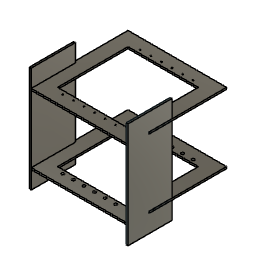
ionenantrieb v1 v1 (Autodesk Fusion 360 design; units mm, degrees)
Autodesk Fusion 360 part; units mm, degrees
sketch "Skizze1" plane through (0, 0, 0) normal (0, 0, 1) x (1, 0, 0)
  line L0 (0, 0) -> (100, 0)
  line L1 (100, 0) -> (100, 100)
  line L2 (100, 100) -> (0, 100)
  line L3 (0, 100) -> (0, 0)
  line L4 (-17.4, -20) -> (120, -20)
  line L5 (120, -20) -> (120, 120)
  line L6 (120, 120) -> (-20, 120)
  line L7 (-20, 120) -> (-20, 10)
  line L8 (-20, 10) -> (-17.4, 10)
  line L9 (-17.4, 10) -> (-17.4, -20)
  line L10 (50, 0) -> (50, 5)
  line L11 (117.4, 10) -> (117.4, -20)
  line L12 (120, 10) -> (117.4, 10)
  dimension "d1" = 100
  dimension "d2" = 100
  dimension "d4" = 2.6
  dimension "d5" = 30
  constraint horizontal L0
  constraint vertical L1
  constraint horizontal L2
  constraint vertical L3
  constraint coincident L0.start L3.end
  constraint perpendicular L7 L8
  constraint perpendicular L4 L9
  constraint parallel L0 L4
  constraint parallel L1 L5
  constraint parallel L2 L6
  constraint parallel L3 L7
  constraint midpoint L0 L10.start
  constraint perpendicular L0 L10
  constraint symmetric L7.end L10 L12.start
  constraint symmetric L8.end L10 L11.start
  constraint symmetric L4.start L10 L11.end
  measures "d1" distance of L1.end L2.end
  measures "d2" distance of L0.start L2.end
  measures "d4" distance of L7.end L8.end
  measures "d5" distance of L8.end L4.start
extrude "Extrusion1" add sketch "Skizze1" along normal blind 2.5 contours L4 L5 L6 L7 L8 L9 L11 L12 makes body 1
sketch "Skizze2" plane through (-17.4, 0, 0) normal (-1, 0, 0) x (0, -1, 0)
  line L0 (-10, 0) -> (20, 0)
  line L1 (20, 0) -> (20, 2.5)
  line L2 (20, 2.5) -> (-10, 2.5)
  line L3 (-10, 2.5) -> (-10, 0)
  line L4 (20, -25) -> (-42.7296, -25)
  line L5 (-42.7296, 125) -> (20, 125)
  line L6 (20, 125) -> (20, -25)
  line L7 (-10, 2.5) -> (-42.7296, 2.5)
  line L8 (-10, 0) -> (-42.7296, 0)
  line L9 (-10, 0) -> (-10, 2.5)
  line L10 (-42.7296, 50) -> (-35, 50)
  line L11 (-10, 100) -> (-42.7296, 100)
  line L12 (-10, 97.5) -> (-42.7296, 97.5)
  line L13 (-10, 100) -> (-10, 97.5)
  line L14 (-42.7296, -25) -> (-42.7296, 0)
  line L15 (-42.7296, 2.5) -> (-42.7296, 97.5)
  line L16 (-42.7296, 100) -> (-42.7296, 125)
  dimension "d8" = 150
  dimension "d9" = 25
  constraint horizontal L4
  constraint vertical L14
  constraint horizontal L5
  constraint vertical L6
  constraint coincident L2.end L3.start
  constraint coincident L7.end L14
  constraint perpendicular L7 L14
  constraint coincident L0.start L3.end
  constraint perpendicular L8 L14
  constraint perpendicular L10 L14
  constraint symmetric L2.end L10 L12.start
  constraint symmetric L7.end L10 L12.end
  constraint symmetric L0.start L10 L11.start
  constraint symmetric L8.end L10 L11.end
  constraint collinear L14 L15
  constraint coincident L10.start L14
  constraint collinear L15 L16
  measures "d8" distance of L4.end L5.start
  measures "d9" distance of L4 L8
extrude "Extrusion2" add sketch "Skizze2" along normal blind 2.5 separate body makes body 2
ref_plane "Arbeitsebene1" through (-18.65, 11.3648, 50) normal (0, 0, -1) x (0, -1, 0)
mirror "Spiegeln1" about plane through (-18.65, 11.3648, 50) normal (0, 0, -1) of bodies 1 makes body 3
ref_plane "Arbeitsebene2" through (50, 65, 98.75) normal (1, 0, 0) x (0, 1, 0)
mirror "Spiegeln2" about plane through (50, 65, 98.75) normal (1, 0, 0) of bodies 2 makes body 4
sketch "Skizze3" plane through (0, 0, 2.5) normal (0, 0, 1) x (-1, 0, 0)
  line L0 (0, 0) -> (0, -100)
  line L1 (0, -100) -> (-100, -100)
  line L2 (-100, -100) -> (-100, 0)
  line L3 (-100, 0) -> (0, 0)
  line L4 (-120, -120) -> (20, -120)
  line L5 (20, -120) -> (20, -10)
  line L6 (20, -10) -> (17.4, -10)
  line L7 (17.4, -10) -> (17.4, 20)
  line L8 (17.4, 20) -> (-117.4, 20)
  line L9 (-117.4, 20) -> (-117.4, -10)
  line L10 (-117.4, -10) -> (-120, -10)
  line L11 (-120, -10) -> (-120, -120)
  circle A0 centre (-12.5, -105) radius 2
  circle A1 centre (-27.5, -105) radius 2
  circle A2 centre (-42.5, -105) radius 2
  circle A3 centre (-57.5, -105) radius 2
  circle A4 centre (-72.5, -105) radius 2
  line L12 (0, -50) -> (-0.7928, -50)
  circle A5 centre (-27.5, 5) radius 2
  circle A6 centre (-72.5, 5) radius 2
  circle A7 centre (-42.5, 5) radius 2
  circle A8 centre (-57.5, 5) radius 2
  circle A9 centre (-12.5, 5) radius 2
  circle A10 centre (-87.5, -105) radius 2
  circle A11 centre (-87.5, 5) radius 2
  point P0 (-87.5, 5)
  dimension "d16" = 4
  dimension "d17" = 5
  dimension "d18" = 12.5
  dimension "d21" = 75
  dimension "d22" = 0
  constraint midpoint L0 L12.start
  constraint perpendicular L0 L12
  constraint symmetric A0 L12 A9
  constraint symmetric A1 L12 A5
  constraint symmetric A2 L12 A7
  constraint symmetric A3 L12 A8
  constraint symmetric A4 L12 A6
  constraint symmetric L12 A10.centre P0
  constraint symmetric L12 A10 A11
  measures "d16" diameter of A0
  measures "d17" distance of L1 A0.centre
  measures "d18" distance of L0 A0.centre
extrude "Extrusion3" cut sketch "Skizze3" against normal blind 2.5 contours A0 | A1 | A2 | A3 | A4 | A5 | A6 | A7 | A8 | A9 | A10 | A11 bodies 1
sketch "Skizze4" plane through (0, 0, 100) normal (0, 0, 1) x (-1, 0, 0)
  line L0 (0, 0) -> (0, -100)
  line L1 (0, -100) -> (-100, -100)
  line L2 (-100, -100) -> (-100, 0)
  line L3 (-100, 0) -> (0, 0)
  line L4 (-120, -120) -> (20, -120)
  line L5 (20, -120) -> (20, -10)
  line L6 (20, -10) -> (17.4, -10)
  line L7 (17.4, -10) -> (17.4, 20)
  line L8 (17.4, 20) -> (-117.4, 20)
  line L9 (-117.4, 20) -> (-117.4, -10)
  line L10 (-117.4, -10) -> (-120, -10)
  line L11 (-120, -10) -> (-120, -120)
  circle A0 centre (-12.5, -105) radius 1
  circle A1 centre (-27.5, -105) radius 1
  circle A2 centre (-42.5, -105) radius 1
  circle A3 centre (-57.5, -105) radius 1
  circle A4 centre (-72.5, -105) radius 1
  line L12 (0, -50) -> (-0.625, -50)
  circle A5 centre (-27.5, 5) radius 1
  circle A6 centre (-72.5, 5) radius 1
  circle A7 centre (-42.5, 5) radius 1
  circle A8 centre (-12.5, 5) radius 1
  circle A9 centre (-57.5, 5) radius 1
  circle A10 centre (-87.5, -105) radius 1
  circle A11 centre (-87.5, 5) radius 1
  dimension "d25" = 2
  dimension "d26" = 5
  dimension "d27" = 12.5
  dimension "d30" = 75
  dimension "d31" = 0
  constraint midpoint L0 L12.start
  constraint perpendicular L0 L12
  constraint symmetric A0 L12 A8
  constraint symmetric A1 L12 A5
  constraint symmetric A2 L12 A7
  constraint symmetric A3 L12 A9
  constraint symmetric A4 L12 A6
  constraint symmetric L12 A10 A11
  measures "d25" diameter of A0
  measures "d26" distance of L1 A0.centre
  measures "d27" distance of L0 A0.centre
extrude "Extrusion4" cut sketch "Skizze4" against normal blind 2.5 contours A0 | A1 | A2 | A3 | A4 | A5 | A6 | A7 | A8 | A9 | A10 | A11 bodies 3
sketch "Skizze5" plane through (117.4, 0, 0) normal (-1, 0, 0) x (0, -1, 0)
  line L0 (-10, 100) -> (-10, 97.5)
  line L1 (-10, 97.5) -> (-42.7296, 97.5)
  line L2 (-42.7296, 97.5) -> (-42.7296, 2.5)
  line L3 (-42.7296, 2.5) -> (-10, 2.5)
  line L4 (-10, 2.5) -> (-10, 0)
  line L5 (-10, 0) -> (-42.7296, 0)
  line L6 (-42.7296, 0) -> (-42.7296, -25)
  line L7 (-42.7296, -25) -> (20, -25)
  line L8 (20, -25) -> (20, 125)
  line L9 (20, 125) -> (-42.7296, 125)
  line L10 (-42.7296, 125) -> (-42.7296, 100)
  line L11 (-42.7296, 100) -> (-10, 100)
equation "d18 = ( 100 / 8 ) * 1 mm"
equation "d21 = 100 mm - ( 2 * 100 / 8 ) * 1 mm"
equation "d27 = ( 100 / 8 ) * 1 mm"
equation "d30 = 100 mm - ( 2 * 100 / 8 ) * 1 mm"
